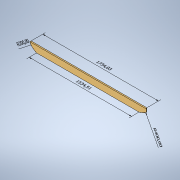
# Autodesk Inventor part: HolzPlatterechts
Saved by Autodesk Inventor 2020.3 (Build 243373010, 373A)
## iProperties
Created: 2021-02-05
Part Number: HolzPlatterechts
Material: Generisch
Document SubType Name: Modeling
Designer: Stefan
Density: 1 g/cm^3
Appearance: Fichte
Author: Stefan
Autodesk Inventor part; units mm, degrees
ref_plane "YZ Plane" through (0, 0, 0) normal (1, 0, 0) x (0, 1, 0)
ref_plane "XZ Plane" through (0, 0, 0) normal (0, 1, 0) x (-1, 0, 0)
ref_plane "XY Plane" through (0, 0, 0) normal (0, 0, 1) x (1, 0, 0)
sketch "Skizze1" plane through (0, 0, 0) normal (0, 0, 1) x (1, 0, 0)
  line L0 (-3157.2887, 244.4054) -> (-1410.3053, 244.4054)
  line L1 (-1410.3053, 199.2768) -> (-1410.3053, 244.4054)
  arc A0 (-1520.1704, 149.4054) -> (-1410.3053, 199.2768) centre (-1628.683, 534.4054) ccw
  line L2 (-3054.6765, 149.4054) -> (-1520.1704, 149.4054)
  arc A1 (-3157.2887, 244.4054) -> (-3054.6765, 149.4054) centre (-2978.683, 334.4054) ccw
  point P0 (-2370.1189, 0)
  point P1 (-1410.3053, 199.2768)
  point P2 (-1410.3053, 244.4054)
  dimension "d59" = 400
  dimension "d60" = 200
  dimension "d61" = 95
  dimension "d62" = 0
  dimension "d63" = 0
  dimension "d64" = 45.1286
  dimension "d65" = 0
  dimension "d66" = 45.1286
  dimension "d67" = 109.865
  dimension "d68" = 109.865
  dimension "d69" = 95
  dimension "d70" = 959.8136
  dimension "d71" = 244.4054
  dimension "d72" = 1568.3777
  dimension "d73" = 90
  dimension "d74" = 1644.3711
  dimension "d75" = 1644.3711
  dimension "d76" = 1746.9834
  dimension "d77" = 1746.9834
  constraints: 6 end point, 4 point on circle, 2 centre point, 1 horizontal, 1 parallel, 1 vertical
  measures "d59" radius of A0
  measures "d60" radius of A1
  measures "d61" distance between parallel lines of L0 L2
  measures "d62" distance from line of L0.end L1
  measures "d63" distance from line of L1.end L0
  measures "d64" distance from line of L1.start L0
  measures "d65" distance from line of A0.end L1
  measures "d66" distance from line of A0.end L0
  measures "d67" distance from line of L2.end L1
  measures "d68" distance from line of A0.start L1
  measures "d69" distance from line of A0.start L0
  measures "d70" distance from line of point (-2370.119, 0) L1
  measures "d71" distance from line of point (-2370.119, 0) L0
  measures "d72" distance from line of A1.centre L1
  measures "d73" distance from line of A1.centre L0
  measures "d74" distance from line of L2.start L1
  measures "d75" distance from line of A1.end L1
  measures "d76" distance from line of L0.start L1
  measures "d77" distance from line of A1.start L1
extrude "Extrusion1" add sketch "Skizze1" along normal blind 20
sketch "Skizze2" plane through (-3157.2887, 244.4054, 0) normal (0, 1, 0) x (1, 0, 0)
  line L0 (1746.9834, -20) -> (1856.261, -20)
  ellipse E0 centre (1857.974, 0) end of major axis (1731.8988, 18.1709) minor radius 65.6716 (1734.0318, 0) -> (1746.9834, -20) ccw
  line L1 (1746.9834, 0) -> (0, 0) projected
  line L2 (1746.9834, 0) -> (1746.9834, -20) projected
  line L3 (1856.261, -20) -> (1856.261, 0)
  line L4 (1856.261, 0) -> (1734.0318, 0)
  line L5 (1637.1184, 0) -> (1746.9834, 0) projected
  point P0 (3157.2887, 0)
  point P1 (1734.0318, 0)
  dimension "d59" = 400
  dimension "d87" = 0
  dimension "d88" = 109.2776
  constraints: 6 end point, 1 collinear, 1 vertical, 5 other
  measures "d87" distance from line of L2 L0.start
  measures "d88" distance of L0.start L0.end
extrude "Extrusion2" cut sketch "Skizze2" against normal through all
